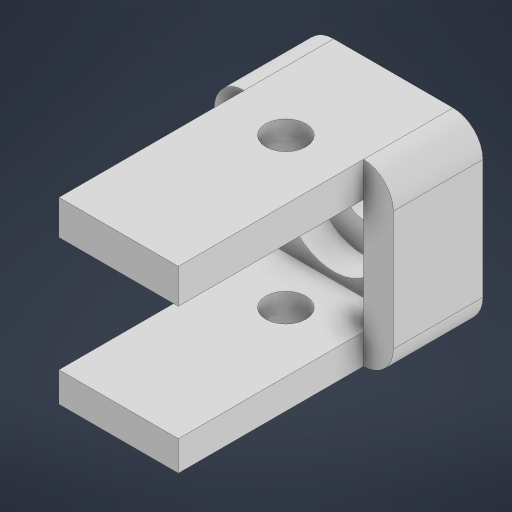
# Autodesk Inventor part: pto piston part
Saved by Autodesk Inventor 2024 (Build 280153000, 153)
## iProperties
Created: 2024-03-30
Part Number: pto piston part
Material: Generic
Document SubType Name: Modeling
Designer: Andrew
Density: 1 g/cm^3
Appearance: Default
Author: Andrew
Autodesk Inventor part; units mm, degrees
ref_plane "YZ Plane" through (0, 0, 0) normal (1, 0, 0) x (0, 1, 0)
ref_plane "XZ Plane" through (0, 0, 0) normal (0, 1, 0) x (-1, 0, 0)
ref_plane "XY Plane" through (0, 0, 0) normal (0, 0, 1) x (1, 0, 0)
sketch "Sketch1" plane through (0, 0, 0) normal (1, 0, 0) x (0, 1, 0)
  line L0 (-5.834, -11.9665) -> (6.358, -11.9665)
  line L1 (6.358, -11.9665) -> (9.533, -11.9665)
  line L2 (-5.834, -11.9665) -> (-9.009, -11.9665)
  line L3 (6.358, -11.9665) -> (10.041, -11.9665)
  line L4 (10.041, -11.9665) -> (10.041, 10.8935)
  line L5 (10.041, 10.8935) -> (6.358, 10.8935)
  line L6 (6.358, 10.8935) -> (6.358, -11.9665)
  line L7 (-9.009, -11.9665) -> (-5.834, -11.9665)
  line L8 (-5.834, -11.9665) -> (-5.834, 10.8935)
  line L9 (-5.834, 10.8935) -> (-9.009, 10.8935)
  line L10 (-9.009, 10.8935) -> (-9.009, -11.9665)
  line L11 (10.041, -11.9665) -> (-9.009, -11.9665)
  line L12 (-9.009, -11.9665) -> (-9.009, -18.3165)
  line L13 (-9.009, -18.3165) -> (10.041, -18.3165)
  line L14 (10.041, -18.3165) -> (10.041, -11.9665)
  point P0 (0, 0)
  dimension "d0" = 12.192
  dimension "d1" = 3.175
  dimension "d2" = 3.175
  dimension "d3" = 22.86
  constraints: 30 end point, 6 horizontal, 6 parallel, 3 perpendicular
  measures "d0" distance of L0.start L0.end
  measures "d1" distance of L0.end L1.end
  measures "d2" distance of L0.start L2.end
  measures "d3" distance of L3.end L4.end
extrude "Extrusion1" add sketch "Sketch1" along normal blind 12.7
sketch "Sketch2" plane through (0, -5.834, 10.8935) normal (0, 1, 0) x (1, 0, 0)
  line L0 (0, 22.86) -> (12.7, 22.86) projected
  line L1 (12.7, 22.86) -> (0, 22.86)
  line L2 (6.35, 22.86) -> (6.35, 17.78)
  circle A0 centre (6.35, 17.78) radius 2.1336
  point P0 (0, 10.8935)
  dimension "d6" = 5.08
  dimension "d7" = 4.2672
  constraints: 4 end point, 1 centre point, 1 coincident, 1 collinear, 1 midpoint, 1 vertical
  measures "d6" distance of L2.start L2.end
  measures "d7" diameter of A0
extrude "Extrusion2" cut sketch "Sketch2" along normal through all both and the other way through all
sketch "Sketch3" plane through (12.7, 0, 0) normal (1, 0, 0) x (0, 0, -1)
  line L0 (18.3165, 10.041) -> (-10.8935, 10.041) projected
  line L1 (11.9665, 6.358) -> (11.9665, -5.834) projected
  line L2 (-10.8935, -9.009) -> (18.3165, -9.009) projected
  line L3 (18.3165, -9.009) -> (18.3165, 10.041) projected
  line L4 (18.3165, 10.041) -> (11.9665, 10.041)
  line L5 (11.9665, 10.041) -> (11.9665, -9.009)
  line L6 (11.9665, -9.009) -> (18.3165, -9.009)
  line L7 (18.3165, -9.009) -> (18.3165, 10.041)
  point P0 (0, 0)
  point P1 (11.9665, -5.834)
  point P2 (11.9665, 6.358)
  constraints: 8 end point, 2 parallel, 1 horizontal, 1 perpendicular, 1 point on line
extrude "Extrusion3" add sketch "Sketch3" along normal blind 3.175
sketch "Sketch4" plane through (0, 0, 0) normal (-1, 0, 0) x (0, 0, 1)
  line L0 (-18.3165, 10.041) -> (10.8935, 10.041) projected
  line L1 (-18.3165, -9.009) -> (-18.3165, 10.041) projected
  line L2 (10.8935, -9.009) -> (-18.3165, -9.009) projected
  line L3 (-11.9665, 6.358) -> (-11.9665, -5.834) projected
  line L4 (-11.9665, 6.358) -> (-11.9665, 10.041) projected
  line L5 (-18.3165, -9.009) -> (-11.9665, -9.009)
  line L6 (-11.9665, -9.009) -> (-11.9665, 10.041)
  line L7 (-11.9665, 10.041) -> (-18.3165, 10.041)
  line L8 (-18.3165, 10.041) -> (-18.3165, -9.009)
  point P0 (0, 0)
  constraints: 8 end point, 2 parallel, 1 horizontal, 1 perpendicular
extrude "Extrusion4" add sketch "Sketch4" along normal blind 3.175
sketch "Sketch5" plane through (0, -5.834, -11.9665) normal (0, 0, 1) x (1, 0, 0)
  line L0 (12.7, -3.175) -> (12.7, 0) projected
  line L1 (12.7, -3.175) -> (15.875, -3.175) projected
  line L2 (15.875, 15.875) -> (15.875, -3.175) projected
  line L3 (12.7, 15.875) -> (15.875, 15.875) projected
  line L4 (12.7, 12.192) -> (12.7, 15.875) projected
  line L5 (0, 15.875) -> (0, 12.192) projected
  line L6 (0, 15.875) -> (-3.175, 15.875) projected
  line L7 (-3.175, -3.175) -> (-3.175, 15.875) projected
  line L8 (0, -3.175) -> (-3.175, -3.175) projected
  line L9 (0, 0) -> (0, -3.175) projected
  line L10 (-3.175, 15.875) -> (0, 15.875)
  line L11 (0, 15.875) -> (0, -3.175)
  line L12 (0, -3.175) -> (-3.175, -3.175)
  line L13 (-3.175, -3.175) -> (-3.175, 15.875)
  line L14 (12.7, -3.175) -> (15.875, -3.175)
  line L15 (15.875, -3.175) -> (15.875, 15.875)
  line L16 (15.875, 15.875) -> (12.7, 15.875)
  line L17 (12.7, 15.875) -> (12.7, -3.175)
  point P0 (0, 5.834)
  constraints: 16 end point, 4 parallel, 2 horizontal, 2 perpendicular
extrude "Extrusion5" add sketch "Sketch5" along normal blind 3.175
sketch "Sketch6" plane through (0, 6.358, -11.9665) normal (0, 0, 1) x (1, 0, 0)
  line L0 (0, 0) -> (12.7, 0) projected
  line L1 (0, -12.192) -> (12.7, -12.192) projected
  line L2 (6.35, 0) -> (6.35, -12.192)
  circle A0 centre (6.35, -6.096) radius 5.334
  point P0 (0, -6.358)
  dimension "d16" = 10.668
  constraints: 3 midpoint, 2 end point, 1 centre point
  measures "d16" diameter of A0
extrude "Extrusion6" cut sketch "Sketch6" against normal blind 3.175
sketch "Sketch7" plane through (6.35, 0.262, -15.1415) normal (0, 0, 1) x (1, 0, 0)
  circle A0 centre (0, 0) radius 5.334 projected
  circle A1 centre (0, 0) radius 2.1336
  point P0 (-6.35, -0.262)
  dimension "d19" = 4.2672
  constraints: 1 centre point, 1 coincident
  measures "d19" diameter of A1
extrude "Extrusion7" cut sketch "Sketch7" against normal through all contours A1
fillet "Fillet1" radius 3.175 4 edges at (15.875, -9.009, -13.554) (15.875, 10.041, -13.554) (-3.175, 10.041, -13.554) (-3.175, -9.009, -13.554)
body "Solid1"
